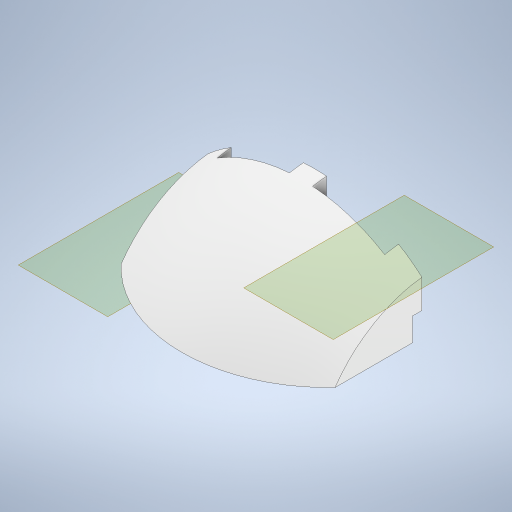
# Autodesk Inventor part: body back for main 3
Saved by Autodesk Inventor 2023 (Build 270158000, 158)
## iProperties
Created: 2022-10-08
Part Number: body back for main 3
Material: ABS プラスチック
Document SubType Name: Modeling
Designer: ellie
Density: 1.06 g/cm^3
Appearance: 積雪
Author: ellie
Autodesk Inventor part; units mm, degrees
ref_plane "YZ Plane" through (0, 0, 0) normal (1, 0, 0) x (0, 1, 0)
sketch "スケッチ1" plane through (0, 0, 0) normal (0, 1, 0) x (-1, 0, 0)
  circle A0 centre (0, 0) radius 35
  line L0 (0, 0) -> (0, -35)
  line L1 (0, 0) -> (0, 35)
  dimension "d0" = 70
  constraints: 4 end point, 2 point on circle, 2 vertical, 1 centre point, 1 coincident
  measures "d0" diameter of A0
revolve "回転1" add sketch "スケッチ1" angle 180 about axis through (0, 0, 0) along (0, 0, 1) picked at (-2.5961, -23.0408) contours L1 L0 A0
sketch "スケッチ5" plane through (0, 0, 0) normal (0, -1, 0) x (1, 0, 0)
  line L0 (-20, -23) -> (20, -23)
  line L1 (20, -23) -> (20, -13)
  line L2 (20, -13) -> (-20, -13)
  line L3 (-20, -13) -> (-20, -23)
  line L4 (-20, -15) -> (-20, -13)
  line L5 (0, 25) -> (-17, 25)
  line L6 (-17, 25) -> (-17, 23)
  line L7 (-17, 23) -> (0, 23)
  line L8 (0, 23) -> (0, 25)
  line L9 (0, 20) -> (-20, 20)
  line L10 (-20, 20) -> (-20, 19)
  line L11 (-20, 19) -> (0, 19)
  line L12 (0, 19) -> (0, 20)
  line L13 (0, 13) -> (-19, 13)
  line L14 (-19, 13) -> (-19, 11)
  line L15 (-19, 11) -> (0, 11)
  line L16 (0, 11) -> (0, 13)
  line L17 (0, 5) -> (-23, 5)
  line L18 (-23, 5) -> (-23, 3)
  line L19 (-23, 3) -> (0, 3)
  line L20 (0, 3) -> (0, 5)
  circle A0 centre (0, 0) radius 35 projected
  circle A1 centre (0, 0) radius 35 projected
  line L21 (0, 35) -> (0, -35)
  line L22 (35, 0) -> (-35, 0)
  line L23 (-32, 2) -> (-23, 2)
  line L24 (-23, 2) -> (-23, -8)
  line L25 (-23, -8) -> (-32, -8)
  line L26 (-32, -8) -> (-32, 2)
  line L27 (-23, -8.0262) -> (-23, 2)
  line L28 (-27, 22.2711) -> (-27, -22.2711)
  line L29 (-15.5, 25) -> (0, 25)
  line L30 (0, 25) -> (0, 35)
  line L31 (0, 35) -> (-15.5, 35)
  line L32 (-15.5, 35) -> (-15.5, 25)
  line L33 (-15.5, 23) -> (0, 23)
  line L34 (0, 23) -> (0, 20)
  line L35 (0, 20) -> (-15.5, 20)
  line L36 (-15.5, 20) -> (-15.5, 23)
  line L37 (-16, 13) -> (0, 13)
  line L38 (0, 13) -> (0, 19)
  line L39 (0, 19) -> (-16, 19)
  line L40 (-16, 19) -> (-16, 13)
  line L41 (-16, 11) -> (0, 11)
  line L42 (0, 11) -> (0, 5)
  line L43 (0, 5) -> (-16, 5)
  line L44 (-16, 5) -> (-16, 11)
  line L45 (-23, -3) -> (-39.6865, -3)
  line L46 (-23, -3) -> (-7.8337, -3)
  line L47 (-8, 3) -> (-23, 3)
  line L48 (-23, 3) -> (-23, -9)
  line L49 (-23, -9) -> (-8, -9)
  line L50 (-8, -9) -> (-8, 3)
  line L51 (-8, 3) -> (-23, -9) construction
  line L52 (-23, 3) -> (-8, -9) construction
  line L53 (-23, 4) -> (-33, 4)
  line L54 (-33, 4) -> (-33, -10)
  line L55 (-33, -10) -> (-23, -10)
  line L56 (-23, -10) -> (-23, 4)
  line L57 (-23, 4) -> (-33, -10) construction
  line L58 (-33, 4) -> (-23, -10) construction
  line L59 (-8, 3) -> (-1, 3)
  line L60 (-1, 3) -> (-1, -9)
  line L61 (-1, -9) -> (-8, -9)
  line L62 (-8, -9) -> (-8, 3)
  line L63 (-8, 3) -> (-1, -9) construction
  line L64 (-1, 3) -> (-8, -9) construction
  line L65 (-23, 2) -> (-27, 2)
  line L66 (-23, -8) -> (-27, -8)
  line L67 (-23, 4) -> (-27, 4)
  line L68 (-23, -10) -> (-27, -10)
  line L69 (23.4307, -26) -> (-23.4307, -26)
  line L70 (-8, 3) -> (-6.8, 3)
  line L71 (-6.8, 3) -> (-6.8, -9)
  line L72 (-6.8, -9) -> (-8, -9)
  line L73 (-8, -9) -> (-8, 3)
  line L74 (-3, 5) -> (0, 5)
  line L75 (0, 20) -> (-4, 20)
  line L76 (-4, 19) -> (0, 19)
  line L77 (0, 19) -> (0, 20)
  line L78 (-6, 5) -> (-1, 5)
  line L79 (-1, 3) -> (-6, 3)
  point P0 (0, -23)
  point P1 (0, -13)
  point P2 (0, 24)
  point P3 (0, 19.5)
  point P4 (0, 12)
  point P5 (0, 4)
  point P6 (-20, -18)
  point P7 (-27, -0.5262)
  point P8 (-27, -8)
  point P9 (-15.5, 21.5)
  point P10 (-15.5, 31.3807)
  point P11 (0, 25)
  point P12 (0, 23)
  point P13 (0, 11)
  point P14 (0, 13)
  point P15 (-27, 0)
  point P16 (-32, 0)
  point P17 (-23, 0)
  point P18 (-15.5, -3)
  point P19 (-28, -3)
  point P20 (-4.5, -3)
  point P21 (-8, -9)
  point P22 (-8, 3)
  point P23 (-27, 0.5)
  point P24 (-28, 0.4738)
  point P25 (-28, -11.5262)
  point P26 (-27, -11.5)
  point P27 (-23, 2)
  point P28 (-23, 2)
  point P29 (-8, 0)
  point P30 (-1, 0)
  point P31 (0, 19)
  point P32 (0, 20)
  point P33 (-27, -10)
  point P34 (-27, 4)
  dimension "d12" = 40
  dimension "d13" = 10
  dimension "d23" = 17
  dimension "d24" = 2
  dimension "d27" = 20
  dimension "d28" = 1
  dimension "d30" = 19
  dimension "d31" = 2
  dimension "d33" = 2
  dimension "d88" = 0
  dimension "d89" = 0
  dimension "d90" = 12
  dimension "d92" = 20
  dimension "d93" = 10
  dimension "d97" = 9
  dimension "d98" = 10
  dimension "d113" = 27
  dimension "d122" = 15.5
  dimension "d123" = 35
  dimension "d124" = 3
  dimension "d125" = 15.5
  dimension "d126" = 6
  dimension "d127" = 6
  dimension "d128" = 16
  dimension "d129" = 16
  dimension "d147" = 12
  dimension "d149" = 8
  dimension "d151" = 15
  dimension "d161" = 14
  dimension "d162" = 10
  dimension "d164" = 12
  dimension "d165" = 7
  dimension "d170" = 26
  dimension "d175" = 1.2
  dimension "d207" = 0
  constraints: 158 end point, 31 parallel, 20 horizontal, 17 perpendicular, 16 point on line, 15 midpoint, 10 collinear, 1 vertical, 20 other
  measures "d12" distance of L2.end L1.end
  measures "d13" distance of L1.end L0.end
  measures "d23" distance of L7.end L6.end
  measures "d24" distance of L6.end L5.end
  measures "d27" distance of L11.end L10.end
  measures "d28" distance of L10.end L9.end
  measures "d30" distance of L15.end L14.end
  measures "d31" distance of L14.end L13.end
  measures "d33" distance of L18.end L17.end
  measures "d89" distance from line of point (0, 0) L22
  measures "d90" distance from line of L0 point (0, -35)
  measures "d92" distance of the line from the sketch origin of L3
  measures "d93" distance from line of L5 point (0, 35)
  measures "d97" distance of L24.end L25.end
  measures "d98" distance of L23.end L24.end
  measures "d113" distance of the line from the sketch origin of L28
  measures "d122" distance of the line from the sketch origin of L32
  measures "d123" distance between parallel lines of L31 L22
  measures "d124" distance of L33.end L34.end
  measures "d126" distance of L38.end L37.end
  measures "d127" distance of L41.end L42.end
  measures "d128" distance of the line from the sketch origin of L44
  measures "d129" distance of the line from the sketch origin of L40
  measures "d147" distance of L48.end L47.end
  measures "d149" distance of the line from the sketch origin of L50
  measures "d151" distance between parallel lines of L50 L24
  measures "d161" distance between parallel lines of L55 L53
  measures "d162" distance between parallel lines of L48 L54
  measures "d164" distance between parallel lines of L61 L59
  measures "d165" distance between parallel lines of L50 L60
  measures "d170" distance between parallel lines of L69 L22
  measures "d175" distance of L71.end L72.end
  measures "d207" distance between parallel lines of L47 L19
extrude "GNSボード" cut sketch "スケッチ5" against normal blind 16 contours L8 L7 L6 L5
extrude "GNSボード止めるよう" cut sketch "スケッチ5" against normal blind 15 contours L21 L5 L32 A0 | L21 L9 L36 L7
extrude "アルミ板１" cut sketch "スケッチ5" against normal blind 20 contours L11 L10 L9 L12
extrude "メイン基板" cut sketch "スケッチ5" against normal blind 17.5 contours L15 L14 L13 L16
extrude "メイン止めるよう" cut sketch "スケッチ5" against normal blind 14.5 contours L17 L44 L15 L21 | L13 L40 L11 L21
extrude "アルミ板２" cut sketch "スケッチ5" against normal blind 20 contours L19 L18 L17 L20
extrude "電池ボックス入れ" cut sketch "スケッチ5" against normal blind 13 contours L3 L2 L21 L0 | L21 L2 L1 L0
extrude "side ut" cut sketch "スケッチ5" against normal blind 100 contours A0 L45 L54 L55 L28 | A0 L22 L54 L45 | L55 L54 L45 L26 L25 L28 | A0 L28 L53 L54 L22 | L54 L22 L26 L45 | L25 L26 L45 L28 | L54 L53 L28 L23 L26 L22 | L26 L22 L28 L45 | L22 L26 L23 L28
extrude "motor case" add sketch "スケッチ5" against normal blind 7 contours L55 L54 L45 L26 L25 L28 | L28 L25 L27 L48 L56 L55 | L50 L46 L24 L22 | L22 L24 L48 L19 L50 | L54 L22 L26 L45 | L28 L45 L24 L25 | L25 L26 L45 L28 | L24 L45 L28 L22 | L22 L28 L23 L24 | L50 L49 L48 L27 L24 L46 | L54 L53 L28 L23 L26 L22 | L26 L22 L28 L45 | L53 L18 L48 L23 L28 | L22 L26 L23 L28
extrude "bottom cut" cut sketch "スケッチ5" against normal blind 90 contours L69 A0 L21 | L21 A0 L69
extrude "motor" cut sketch "スケッチ5" against normal blind 6 contours L60 L61 L71 L22 | L22 L71 L19 L60 | L71 L61 L50 L22 | L22 L50 L19 L71 | L50 L46 L24 L22 | L22 L24 L48 L19 L50 | L28 L45 L24 L25 | L25 L26 L45 L28 | L24 L45 L28 L22 | L22 L28 L23 L24 | L50 L49 L48 L27 L24 L46 | L26 L22 L28 L45 | L22 L26 L23 L28
extrude "motor block" add sketch "スケッチ5" against normal blind 10 contours L71 L61 L50 L22 | L22 L50 L19 L71
sketch "スケッチ27" plane through (-33, 0, -10) normal (-1, 0, 0) x (0, 0, 1)
  line L0 (14, 0) -> (0, 0) projected
  circle A0 centre (7, 0) radius 3
  point P0 (10, 0)
  dimension "d198" = 6
  constraints: 1 centre point, 1 midpoint
  measures "d198" diameter of A0
extrude "押し出し36" cut sketch "スケッチ27" against normal blind 27
mirror "ミラー13" about plane through (0, 0, 0) normal (1, 0, 0) of "メイン止めるよう", "メイン基板", "アルミ板１", "GNSボード止めるよう", "GNSボード", "アルミ板２", "motor", "motor case", "押し出し36", "電池ボックス入れ", "side ut", "motor block"
ref_plane "作業平面5" through (-17, 17.5, 23) normal (0, -1, 0) x (1, 0, 0)
ref_plane "作業平面6" through (20, 13, -13) normal (0, 0, -1) x (1, 0, 0)
sketch "スケッチ38" plane through (20, 13, -13) normal (0, 0, -1) x (1, 0, 0)
  line L0 (-40, 13) -> (0, 13) projected
  line L1 (-40, 13) -> (-40, 0) projected
  line L2 (-40, 0) -> (0, 0) projected
  line L3 (0, 13) -> (0, 0) projected
  line L4 (-38, 6) -> (-28, 6)
  line L5 (-28, 6) -> (-28, -3)
  line L6 (-28, -3) -> (-38, -3)
  line L7 (-38, -3) -> (-38, 6)
  point P0 (-20, 13)
  dimension "d235" = 3
  dimension "d236" = 9
  dimension "d237" = 10
  dimension "d238" = 2
  constraints: 8 end point, 2 parallel, 1 horizontal, 1 perpendicular
  measures "d235" distance between parallel lines of L6 L2
  measures "d236" distance between parallel lines of L6 L4
  measures "d237" distance between parallel lines of L7 L5
  measures "d238" distance between parallel lines of L1 L7
extrude "押し出し44" cut sketch "スケッチ38" against normal blind 18 contours L7 L4 L5 L2 | L2 L5 L6 L7
ref_plane "作業平面7" through (27, 35, 4) normal (0, -1, 0) x (1, 0, 0)
sketch "スケッチ41" plane through (-17, 0, 23) normal (0, -1, 0) x (1, 0, 0)
  line L0 (-16, -23) -> (-15, -23) projected
  line L1 (-15, -23) -> (-15, -21) projected
  line L2 (-15, -21) -> (-6, -21) projected
  line L3 (-6, -21) -> (-6, -18) projected
  line L4 (-6, -18) -> (1, -18) projected
  line L5 (1, -18) -> (1, -12) projected
  line L6 (1, -12) -> (-2, -12) projected
  line L7 (-2, -12) -> (-2, -10) projected
  line L8 (-2, -10) -> (1, -10) projected
  line L9 (1, -10) -> (1, -4) projected
  line L10 (1, -4) -> (-3, -4) projected
  line L11 (-3, -4) -> (-3, -3) projected
  line L12 (-3, -3) -> (1.5, -3) projected
  line L13 (1.5, -3) -> (1.5, 0) projected
  line L14 (1.5, 0) -> (0, 0) projected
  line L15 (0, 0) -> (0, 2) projected
  line L16 (0, 2) -> (1.5, 2) projected
  line L17 (1.5, 2) -> (1.5, 8.3807) projected
  arc A0 (1.5, 8.3807) -> (-10, -0.7289) centre (17, -23) ccw projected
  line L18 (-10, -0.7289) -> (-10, -19) projected
  line L19 (-10, -19) -> (-16, -19) projected
  line L20 (-16, -19) -> (-16, -23) projected
  line L21 (1, -18) -> (1, -12) projected
  line L22 (-2, -10) -> (-2, -12) projected
  line L23 (0, 2) -> (0, 0) projected
  circle A1 centre (-4, 0) radius 2
  dimension "d252" = 4
  dimension "d253" = 4
  dimension "d254" = 3
  constraints: 1 centre point
  measures "d252" diameter of A1
  measures "d253" distance from line of A1.centre L15
  measures "d254" distance from line of A1.centre L12
extrude "押し出し46" cut sketch "スケッチ41" against normal blind 10 contours A1
mirror "ミラー15" about plane through (0, 0, 0) normal (1, 0, 0) of "押し出し46"
sketch "スケッチ42" plane through (-33, 0, -10) normal (0, -1, 0) x (1, 0, 0)
  circle A0 centre (9.5, -8) radius 2
  line L0 (13, -13) -> (13, -3) projected
  line L1 (10, 2) -> (1, 2) projected
  point P0 (33, 10)
  dimension "d257" = 3.5
  dimension "d258" = 4
  dimension "d259" = 10
  constraints: 1 centre point
  measures "d257" distance from line of A0.centre L0
  measures "d258" diameter of A0
  measures "d259" distance from line of A0.centre L1
extrude "押し出し47" cut sketch "スケッチ42" against normal blind 10
mirror "ミラー16" about plane through (0, 0, 0) normal (1, 0, 0) of "押し出し47"
ref_plane "作業平面8" through (-17, 15, 23) normal (0, -1, 0) x (1, 0, 0)
sketch "スケッチ45" plane through (-17, 15, 23) normal (0, -1, 0) x (1, 0, 0)
  circle A0 centre (-4, 0) radius 2 projected
  line L0 (-16, -23) -> (-15, -23) projected
  line L1 (-15, -23) -> (-15, -21) projected
  line L2 (-15, -21) -> (-6, -21) projected
  line L3 (-6, -21) -> (-6, -18) projected
  line L4 (-6, -18) -> (1, -18) projected
  line L5 (1, -18) -> (1, -12) projected
  line L6 (1, -12) -> (-2, -12) projected
  line L7 (-2, -12) -> (-2, -10) projected
  line L8 (-2, -10) -> (1, -10) projected
  line L9 (1, -10) -> (1, -4) projected
  line L10 (1, -4) -> (-3, -4) projected
  line L11 (-3, -4) -> (-3, -3) projected
  line L12 (-3, -3) -> (1.5, -3) projected
  line L13 (1.5, -3) -> (1.5, 0) projected
  line L14 (1.5, 0) -> (0, 0) projected
  line L15 (0, 0) -> (0, 2) projected
  line L16 (0, 2) -> (1.5, 2) projected
  line L17 (1.5, 2) -> (1.5, 8.3807) projected
  arc A1 (1.5, 8.3807) -> (-10, -0.7289) centre (17, -23) ccw projected
  line L18 (-10, -0.7289) -> (-10, -19) projected
  line L19 (-10, -19) -> (-16, -19) projected
  line L20 (-16, -19) -> (-16, -23) projected
  arc A2 (32.5, 4.5636) -> (1.5, 4.5636) centre (17, -23) ccw projected
  line L21 (1.5, 2) -> (1.5, 4.5636) projected
  line L22 (32.5, 2) -> (1.5, 2) projected
  line L23 (32.5, 2) -> (32.5, 4.5636) projected
  circle A3 centre (38, 0) radius 2 projected
  circle A4 centre (38, 0) radius 2 projected
  line L24 (49, -23) -> (50, -23) projected
  line L25 (50, -19) -> (50, -23) projected
  line L26 (44, -19) -> (50, -19) projected
  line L27 (44, -19) -> (44, -0.7289) projected
  arc A5 (44, -0.7289) -> (32.5, 8.3807) centre (17, -23) ccw projected
  line L28 (32.5, 8.3807) -> (32.5, 2) projected
  line L29 (32.5, 2) -> (34, 2) projected
  line L30 (34, 2) -> (34, 0) projected
  line L31 (34, 0) -> (32.5, 0) projected
  line L32 (32.5, 0) -> (32.5, -3) projected
  line L33 (32.5, -3) -> (37, -3) projected
  line L34 (37, -3) -> (37, -4) projected
  line L35 (37, -4) -> (33, -4) projected
  line L36 (33, -4) -> (33, -10) projected
  line L37 (33, -10) -> (36, -10) projected
  line L38 (36, -10) -> (36, -12) projected
  line L39 (36, -12) -> (33, -12) projected
  line L40 (33, -12) -> (33, -18) projected
  line L41 (33, -18) -> (40, -18) projected
  line L42 (40, -18) -> (40, -21) projected
  line L43 (40, -21) -> (49, -21) projected
  line L44 (49, -21) -> (49, -23) projected
  circle A6 centre (-4, 0) radius 2 projected
  line L45 (1.5, 0) -> (32.5, 0) projected
  line L46 (32.5, -3) -> (1.5, -3) projected
  line L47 (32.5, -3) -> (32.5, 0) projected
  line L48 (1.5, 0) -> (32.5, 0) projected
  line L49 (1.5, -3) -> (1.5, 0) projected
  line L50 (34, 0) -> (0, 0) projected
  line L51 (34, 0) -> (34, 2) projected
  line L52 (34, 2) -> (0, 2) projected
  line L53 (0, 0) -> (0, 2) projected
  line L54 (33, -10) -> (1, -10) projected
  line L55 (33, -10) -> (33, -4) projected
  line L56 (1, -4) -> (33, -4) projected
  line L57 (1, -10) -> (1, -4) projected
  line L58 (36, -12) -> (-2, -12) projected
  line L59 (36, -12) -> (36, -10) projected
  line L60 (36, -10) -> (-2, -10) projected
  line L61 (-2, -12) -> (-2, -10) projected
  line L62 (33, -18) -> (1, -18) projected
  line L63 (33, -18) -> (33, -12) projected
  line L64 (1, -12) -> (33, -12) projected
  line L65 (1, -18) -> (1, -12) projected
  line L66 (40, -20) -> (-6, -20) projected
  line L67 (40, -20) -> (40, -18) projected
  line L68 (40, -18) -> (-6, -18) projected
  line L69 (-6, -20) -> (-6, -18) projected
  circle A7 centre (40.5, -41) radius 2 projected
  circle A8 centre (-6.5, -41) radius 2 projected
  line L70 (25, -29) -> (23.8, -29) projected
  line L71 (23.8, -32) -> (23.8, -29) projected
  line L72 (23.8, -32) -> (18, -32) projected
  line L73 (18, -32) -> (18, -20) projected
  line L74 (18, -20) -> (16, -20) projected
  line L75 (16, -20) -> (16, -32) projected
  line L76 (16, -32) -> (10.2, -32) projected
  line L77 (10.2, -32) -> (10.2, -29) projected
  line L78 (10.2, -29) -> (9, -29) projected
  line L79 (9, -29) -> (9, -32) projected
  line L80 (9, -32) -> (-6, -32) projected
  line L81 (-6, -32) -> (-6, -31) projected
  line L82 (-6, -31) -> (-15, -31) projected
  line L83 (-15, -31) -> (-15, -29) projected
  line L84 (-15, -29) -> (-16, -29) projected
  line L85 (-16, -29) -> (-16, -33) projected
  line L86 (-16, -33) -> (-10, -33) projected
  line L87 (-10, -33) -> (-10, -45.2711) projected
  arc A9 (-10, -45.2711) -> (-6.4307, -49) centre (17, -23) ccw projected
  line L88 (-6.4307, -49) -> (40.4307, -49) projected
  arc A10 (40.4307, -49) -> (44, -45.2711) centre (17, -23) ccw projected
  line L89 (44, -45.2711) -> (44, -33) projected
  line L90 (50, -33) -> (44, -33) projected
  line L91 (50, -29) -> (50, -33) projected
  line L92 (50, -29) -> (49, -29) projected
  line L93 (49, -29) -> (49, -31) projected
  line L94 (49, -31) -> (40, -31) projected
  line L95 (40, -31) -> (40, -32) projected
  line L96 (40, -32) -> (25, -32) projected
  line L97 (25, -29) -> (25, -32) projected
  line L98 (-3, -36) -> (37, -36) projected
  line L99 (37, -36) -> (37, -46) projected
  line L100 (37, -46) -> (-3, -46) projected
  line L101 (-3, -46) -> (-3, -36) projected
  line L102 (-6, -18) -> (40, -18)
  line L103 (40, -18) -> (40, 8.6228)
  line L104 (40, 8.6228) -> (-6, 8.6228)
  line L105 (-6, 8.6228) -> (-6, -18)
  arc A11 (32.5, 4.5636) -> (1.5, 4.5636) centre (17, -23) ccw projected
  line L106 (32.5, 4.5636) -> (32.5, 8.3807) projected
  arc A12 (44, -0.7289) -> (32.5, 8.3807) centre (17, -23) ccw projected
  line L107 (44, -0.7289) -> (44, -45.2711) projected
  arc A13 (40.4307, -49) -> (44, -45.2711) centre (17, -23) ccw projected
  line L108 (40.4307, -49) -> (-6.4307, -49) projected
  arc A14 (-10, -45.2711) -> (-6.4307, -49) centre (17, -23) ccw projected
  line L109 (-10, -45.2711) -> (-10, -0.7289) projected
  arc A15 (1.5, 8.3807) -> (-10, -0.7289) centre (17, -23) ccw projected
  line L110 (1.5, 8.3807) -> (1.5, 4.5636) projected
  line L111 (9, -32) -> (9, -20) projected
  line L112 (-6, -20) -> (9, -20) projected
  line L113 (-6, -21) -> (-6, -20) projected
  line L114 (-15, -21) -> (-6, -21) projected
  line L115 (-15, -31) -> (-15, -21) projected
  line L116 (-6, -31) -> (-15, -31) projected
  line L117 (-6, -32) -> (-6, -31) projected
  line L118 (9, -32) -> (-6, -32) projected
  line L119 (50, -29) -> (49, -29) projected
  line L120 (50, -23) -> (50, -29) projected
  line L121 (49, -23) -> (50, -23) projected
  line L122 (49, -29) -> (49, -23) projected
  line L123 (-16, -23) -> (-15, -23) projected
  line L124 (-16, -29) -> (-16, -23) projected
  line L125 (-15, -29) -> (-16, -29) projected
  line L126 (-15, -23) -> (-15, -29) projected
  point P0 (-10, -19)
  point P1 (40, 3.3818)
  point P2 (-6, -20)
  point P3 (-6, -18)
  point P4 (-6, 3.3818)
  point P5 (-10, -31)
  point P6 (44, -31)
  point P7 (-10, -19)
  constraints: 8 end point, 3 collinear, 2 parallel, 1 horizontal, 1 perpendicular, 1 tangent
extrude "side and front cut" cut sketch "スケッチ45" along normal mid plane 100 contours L105 L3 L2 L109 L18 A1 | L66 L111 L79 L80 L81 L82 L109 L2 L3 | L109 L2 L1 L0 L20 L19 | L66 L75 L76 L77 L78 L111 | L109 L82 L83 L115 L1 L2 | L66 L73 L72 L71 L70 L97 L96 L95 L94 L107 L89 A10 L88 A9 L87 L109 L82 L81 L80 L79 L78 L77 L76 L75 | L103 A5 L27 L107 L43 L42 | L0 L115 L84 L124 | L109 L86 L85 L84 L83 L82 | L66 L42 L43 L107 L94 L95 L96 L97 L70 L71 L72 L73 | L26 L25 L24 L44 L43 L107 | L43 L44 L122 L93 L94 L107 | L94 L93 L92 L91 L90 L107 | L120 L92 L122 L24 | A7 | A8 | L98 L99 L100 L101
sketch "スケッチ46" plane through (-17, 15, 23) normal (0, -1, 0) x (1, 0, 0)
  line L0 (-6, 0) -> (-6, -18) projected
  line L1 (-6, -18) -> (1, -18) projected
  line L2 (1, -18) -> (1, -12) projected
  line L3 (1, -12) -> (-2, -12) projected
  line L4 (-2, -12) -> (-2, -10) projected
  line L5 (-2, -10) -> (1, -10) projected
  line L6 (1, -10) -> (1, -4) projected
  line L7 (1, -4) -> (-3, -4) projected
  line L8 (-3, -4) -> (-3, -3) projected
  line L9 (-3, -3) -> (1.5, -3) projected
  line L10 (1.5, -3) -> (1.5, 0) projected
  line L11 (1.5, 0) -> (0, 0) projected
  line L12 (0, 0) -> (0, 2) projected
  line L13 (0, 2) -> (1.5, 2) projected
  line L14 (1.5, 2) -> (1.5, 8.3807) projected
  arc A0 (1.5, 8.3807) -> (-6, 3.3818) centre (17, -23) ccw projected
  line L15 (-6, 3.3818) -> (-6, 0) projected
  circle A1 centre (-4, 0) radius 2 projected
  circle A2 centre (-4, 0) radius 2 projected
  line L16 (40, -18) -> (40, 0) projected
  circle A3 centre (38, 0) radius 2 projected
  line L17 (40, 0) -> (40, 3.3818) projected
  arc A4 (40, 3.3818) -> (32.5, 8.3807) centre (17, -23) ccw projected
  line L18 (32.5, 8.3807) -> (32.5, 2) projected
  line L19 (32.5, 2) -> (34, 2) projected
  line L20 (34, 2) -> (34, 0) projected
  line L21 (34, 0) -> (32.5, 0) projected
  line L22 (32.5, 0) -> (32.5, -3) projected
  line L23 (32.5, -3) -> (37, -3) projected
  line L24 (37, -3) -> (37, -4) projected
  line L25 (37, -4) -> (33, -4) projected
  line L26 (33, -4) -> (33, -10) projected
  line L27 (33, -10) -> (36, -10) projected
  line L28 (36, -10) -> (36, -12) projected
  line L29 (36, -12) -> (33, -12) projected
  line L30 (33, -12) -> (33, -18) projected
  line L31 (33, -18) -> (40, -18) projected
  arc A5 (32.5, 4.5636) -> (1.5, 4.5636) centre (17, -23) ccw projected
  line L32 (1.5, 2) -> (1.5, 4.5636) projected
  line L33 (32.5, 2) -> (1.5, 2) projected
  line L34 (32.5, 2) -> (32.5, 4.5636) projected
  line L35 (34, 0) -> (0, 0) projected
  line L36 (34, 0) -> (34, 2) projected
  line L37 (34, 2) -> (0, 2) projected
  line L38 (0, 0) -> (0, 2) projected
  line L39 (32.5, -3) -> (1.5, -3) projected
  line L40 (32.5, -3) -> (32.5, 0) projected
  line L41 (1.5, 0) -> (32.5, 0) projected
  line L42 (1.5, -3) -> (1.5, 0) projected
  line L43 (33, -10) -> (1, -10) projected
  line L44 (33, -10) -> (33, -4) projected
  line L45 (1, -4) -> (33, -4) projected
  line L46 (1, -10) -> (1, -4) projected
  line L47 (33, -18) -> (1, -18) projected
  line L48 (33, -18) -> (33, -12) projected
  line L49 (1, -12) -> (33, -12) projected
  line L50 (1, -18) -> (1, -12) projected
  point P0 (32.5, 4.5636)
  point P1 (1.5, 4.5636)
  constraints: 3 horizontal alignment
extrude "front cut 2" cut sketch "スケッチ46" along normal blind 100 contours L15 A0 L14 L13 L12 L11 L10 L9 L8 L7 L6 L5 L4 L3 L2 L1 L0 | A1 | L2 L49 L30 L47 | L3 L4 L5 L43 L27 L28 L29 L49 | A3 | L30 L29 L28 L27 L26 L25 L24 L23 L22 L21 L20 L19 L18 A4 L17 L16 L31 | A5 L18 L33 L14 | L33 L19 L20 L21 L35 L11 L12 L13 | L6 L45 L26 L43 | L7 L8 L9 L39 L23 L24 L25 L45 | L35 L22 L39 L10
sketch "スケッチ48" plane through (0, 0, 3) normal (0, 0, -1) x (-1, 0, 0)
  line L0 (-23, 20) -> (23, 20) projected
  line L1 (23, 26.2107) -> (23, 20) projected
  arc A0 (23, 26.2107) -> (-23, 26.2107) centre (0, 0) ccw projected
  line L2 (-23, 26.2107) -> (-23, 20) projected
  line L3 (-23, 15) -> (23, 15) projected
  line L4 (-23, 15) -> (-23, 20) projected
  line L5 (23, 15) -> (23, 20) projected
  line L6 (-23, 40) -> (-18, 40)
  line L7 (-18, 40) -> (-18, 15)
  line L8 (-18, 15) -> (-23, 15)
  line L9 (-23, 15) -> (-23, 40)
  line L10 (18, 40) -> (23, 40)
  line L11 (23, 40) -> (23, 15)
  line L12 (23, 15) -> (18, 15)
  line L13 (18, 15) -> (18, 40)
  line L14 (-2.5, 34.8712) -> (2.5, 34.8712)
  line L15 (2.5, 34.8712) -> (2.5, 20)
  line L16 (2.5, 20) -> (-2.5, 20)
  line L17 (-2.5, 20) -> (-2.5, 34.8712)
  line L18 (0, 0) -> (0, 34.8712)
  point P0 (18, 20)
  point P1 (18, 29.8664)
  point P2 (-18, 29.8664)
  point P3 (-18, 20)
  point P4 (2.5, 34.7815)
  point P5 (2.5, 20)
  point P6 (-2.5, 34.7815)
  dimension "d274" = 25
  dimension "d275" = 5
  dimension "d276" = 25
  dimension "d277" = 5
  dimension "d280" = 5
  dimension "d282" = 2.5
  constraints: 26 end point, 6 parallel, 5 collinear, 3 horizontal, 3 perpendicular, 1 midpoint, 1 point on circle, 1 tangent
  measures "d274" distance between parallel lines of L3 L6
  measures "d275" distance between parallel lines of L9 L7
  measures "d276" distance between parallel lines of L3 L10
  measures "d277" distance between parallel lines of L13 L11
  measures "d280" distance between parallel lines of L17 L15
  measures "d282" distance between parallel lines of L17 L18
extrude "lock cut" cut sketch "スケッチ48" against normal blind 3 contours L7 A0 L17 L0 | L15 A0 L13 L0
